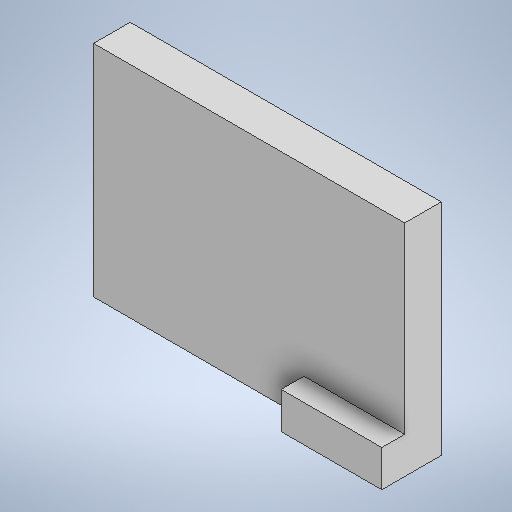
# Autodesk Inventor part: charger
Saved by Autodesk Inventor 2025.3 (Build 293356000, 356)
## iProperties
Created: 2025-06-07
Part Number: charger
Material: Generic
Document SubType Name: Modeling
Designer: Repete
Density: 1 g/cm^3
Appearance: Default
Author: Repete
Autodesk Inventor part; units mm, degrees
ref_plane "YZ Plane" through (0, 0, 0) normal (1, 0, 0) x (0, 1, 0)
ref_plane "XZ Plane" through (0, 0, 0) normal (0, 1, 0) x (-1, 0, 0)
ref_plane "XY Plane" through (0, 0, 0) normal (0, 0, 1) x (1, 0, 0)
sketch "Sketch1" plane through (0, 0, 0) normal (0, 1, 0) x (-1, 0, 0)
  line L0 (15.6279, 8.093) -> (-18.3721, 8.093)
  line L1 (-18.3721, 8.093) -> (-18.3721, -15.907)
  line L2 (-18.3721, -15.907) -> (15.6279, -15.907)
  line L3 (15.6279, -15.907) -> (15.6279, 8.093)
  point P0 (0, 0)
  dimension "d0" = 24
  dimension "d1" = 34
  constraints: 8 end point, 2 parallel, 1 horizontal, 1 perpendicular
  measures "d0" distance of L2.end L0.start
  measures "d1" distance of L1.end L2.end
extrude "Extrusion1" add sketch "Sketch1" along normal blind 4
sketch "Sketch2" plane through (0, 4, 0) normal (0, 1, 0) x (1, 0, 0)
  line L0 (-13.61, -6.4787) -> (16.6862, -6.4787)
  line L1 (16.6862, -6.4787) -> (16.6862, 11.1397)
  line L2 (16.6862, 11.1397) -> (-13.61, 11.1397)
  line L3 (-13.61, 11.1397) -> (-13.61, -6.4787)
  point P0 (0, 0)
  constraints: 8 end point, 2 parallel, 1 horizontal, 1 perpendicular
extrude "Extrusion2" cut sketch "Sketch2" against normal blind 2.5
sketch "Sketch3" plane through (0, 0, 0) normal (0, -1, 0) x (1, 0, 0)
  line L0 (18.3721, -15.907) -> (-15.6279, -15.907) projected
  line L1 (18.3721, -15.907) -> (7.3721, -15.907)
  line L2 (7.3721, -15.907) -> (7.3721, -11.907)
  line L3 (7.3721, -11.907) -> (18.3721, -11.907)
  line L4 (18.3721, -11.907) -> (18.3721, -15.907)
  point P0 (0, 0)
  dimension "d6" = 11
  dimension "d7" = 4
  constraints: 8 end point, 2 parallel, 1 horizontal, 1 perpendicular
  measures "d6" distance of L2.end L3.end
  measures "d7" distance of L1.end L2.end
extrude "Extrusion3" add sketch "Sketch3" along normal blind 2.5
body "Solid1"
